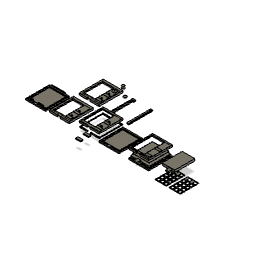
MacroPaw KnGXT (Autodesk Fusion 360 design; units mm, degrees)
Autodesk Fusion 360 part; units mm, degrees
note: some values were not read from the file. Chosen so that the rebuilt part matches the saved one: which bodies a step acts on; which face or edge a step refers to; which pieces of a blend or face edit are solid.
sketch "Sketch1" plane through (0, 0, 0) normal (0, 1, 0) x (1, 0, 0)
  line L0 (-50, -50) -> (44.5, -50)
  line L1 (44.5, -50) -> (44.5, 59)
  line L2 (44.5, 59) -> (-50, 59)
  line L3 (-50, 59) -> (-50, -50)
  dimension "d1" = 94.5
  dimension "d2" = 109
  constraint horizontal L0
  constraint vertical L1
  constraint horizontal L2
  constraint vertical L3
  measures "d1" distance of L0.start L0.end
  measures "d2" distance of L0.start L2.end
extrude "Extrude1" add sketch "Sketch1" along normal blind 1 makes body 1
box "BoxPrimitive1" add length 6 width 15 height 20 placed x (0, 1, 0) y (-1, 0, 0) z (0, 0, 1) at (8.5, 25, 0) separate body makes body 2
move_body "Move1" bodies 2 to x (1, 0, 0) y (0, 1, 0) z (0, 0, 1) at (-3.75, -24, 50)
move_body "Move2" bodies 2 to x (1, 0, 0) y (0, 1, 0) z (0, 0, 1) at (-39.75, 0, 0)
move_body "Move3" bodies 2 to x (1, 0, 0) y (0, 1, 0) z (0, 0, 1) at (35, -1, 0)
copy_body "CopyPasteBodies1" bodies 1 makes body 3
move_body "Move4" bodies 3 to x (1, 0, 0) y (0, 1, 0) z (0, 0, 1) at (0, -10, 0)
copy_body "CopyPasteBodies2" bodies 3 makes body 4
move_body "Move5" bodies 4 to x (1, 0, 0) y (0, 1, 0) z (0, 0, 1) at (0, -10, 0)
move_face "OffsetFaces1" offset -5 1 faces at (-50, -9.6667, -22.6667) on bodies 3
move_face "OffsetFaces2" offset -3 1 faces at (-15.1667, -9.3333, -59) on bodies 3
move_face "OffsetFaces3" offset -5 1 faces at (44.5, -9.3333, -20.6667) on bodies 3
move_face "OffsetFaces4" offset -5 1 faces at (-16.8333, -9.6667, 50) on bodies 3
copy_body "CopyPasteBodies3" bodies 3 makes body 5
move_body "Move6" bodies 5 to x (1, 0, 0) y (0, 1, 0) z (0, 0, 1) at (0, 20, 0)
move_face "OffsetFaces5" offset 3 1 faces at (-16.8333, -10, -22.3333) on bodies 3
copy_body "CopyPasteBodies4" bodies 1 makes body 6
move_body "Move7" bodies 6 to x (1, 0, 0) y (0, 1, 0) z (0, 0, 1) at (0, -10, 0)
move_face "OffsetFaces6" offset 5 1 faces at (13, -19.6667, -59) on bodies 4
move_face "OffsetFaces7" offset 5 1 faces at (-18.5, -19.6667, 50) on bodies 4
move_face "OffsetFaces8" offset 5 1 faces at (-18.5, -19, -24.3333) on bodies 4
move_body "Move8" bodies 4 to x (1, 0, 0) y (0, 1, 0) z (0, 0, 1) at (0, 5, 0)
copy_body "CopyPasteBodies5" bodies 2 makes body 7
move_body "Move9" bodies 7 to x (1, 0, 0) y (0, 1, 0) z (0, 0, 1) at (0, -10, 0)
combine "Combine1" operation cut target body 4 tool bodies 3 6 7
sketch "Sketch3" plane through (0, 1, 0) normal (0, 1, 0) x (-1, 0, 0)
  line L0 (50, -59) -> (50, 50)
  line L1 (50, 50) -> (-44.5, 50)
  line L2 (-44.5, 50) -> (-44.5, -59)
  line L3 (-44.5, -59) -> (50, -59)
  line L4 (-175, 0) -> (-118.9, 0)
  line L5 (-118.9, 0) -> (-118.9, 94.2)
  line L6 (-118.9, 94.2) -> (-175, 94.2)
  line L7 (-175, 94.2) -> (-175, 0)
  dimension "d39" = 56.1
  dimension "d40" = 94.2
  constraint horizontal L4
  constraint vertical L5
  constraint horizontal L6
  constraint vertical L7
  measures "d39" distance of L4.start L4.end
  measures "d40" distance of L4.start L6.end
sketch "Sketch4" plane through (0, 11, 0) normal (0, 1, 0) x (-1, 0, 0)
  line L0 (45, -56) -> (45, 45)
  line L1 (45, 45) -> (-39.5, 45)
  line L2 (-39.5, 45) -> (-39.5, -56)
  line L3 (-39.5, -56) -> (45, -56)
  line L4 (-173, 2) -> (-159, 2)
  line L5 (-159, 2) -> (-159, 16)
  line L6 (-159, 16) -> (-173, 16)
  line L7 (-173, 16) -> (-173, 2)
  line L8 (-173, 21.05) -> (-159, 21.05)
  line L9 (-159, 21.05) -> (-159, 35.05)
  line L10 (-159, 35.05) -> (-173, 35.05)
  line L11 (-173, 35.05) -> (-173, 21.05)
  line L12 (-173, 40.1) -> (-159, 40.1)
  line L13 (-159, 40.1) -> (-159, 54.1)
  line L14 (-159, 54.1) -> (-173, 54.1)
  line L15 (-173, 54.1) -> (-173, 40.1)
  line L16 (-173, 59.15) -> (-159, 59.15)
  line L17 (-159, 59.15) -> (-159, 73.15)
  line L18 (-159, 73.15) -> (-173, 73.15)
  line L19 (-173, 73.15) -> (-173, 59.15)
  line L20 (-173, 78.2) -> (-159, 78.2)
  line L21 (-159, 78.2) -> (-159, 92.2)
  line L22 (-159, 92.2) -> (-173, 92.2)
  line L23 (-173, 92.2) -> (-173, 78.2)
  line L24 (-118.9, 94.2) -> (-175, 94.2)
  line L25 (-153.95, 78) -> (-139.95, 78)
  line L26 (-139.95, 78) -> (-139.95, 92)
  line L27 (-139.95, 92) -> (-153.95, 92)
  line L28 (-153.95, 92) -> (-153.95, 78)
  line L29 (-153.95, 59) -> (-139.95, 59)
  line L30 (-139.95, 59) -> (-139.95, 73)
  line L31 (-139.95, 73) -> (-153.95, 73)
  line L32 (-153.95, 73) -> (-153.95, 59)
  line L33 (-153.95, 40) -> (-139.95, 40)
  line L34 (-139.95, 40) -> (-139.95, 54)
  line L35 (-139.95, 54) -> (-153.95, 54)
  line L36 (-153.95, 54) -> (-153.95, 40)
  line L37 (-153.95, 21) -> (-139.95, 21)
  line L38 (-139.95, 21) -> (-139.95, 35)
  line L39 (-139.95, 35) -> (-153.95, 35)
  line L40 (-153.95, 35) -> (-153.95, 21)
  line L41 (-144.425, 2) -> (-130.425, 2)
  line L42 (-130.425, 2) -> (-130.425, 16)
  line L43 (-130.425, 16) -> (-144.425, 16)
  line L44 (-144.425, 16) -> (-144.425, 2)
  line L45 (-134.9, 78) -> (-120.9, 78)
  line L46 (-120.9, 78) -> (-120.9, 92)
  line L47 (-120.9, 92) -> (-134.9, 92)
  line L48 (-134.9, 92) -> (-134.9, 78)
  line L49 (-134.9, 59) -> (-120.9, 59)
  line L50 (-120.9, 59) -> (-120.9, 73)
  line L51 (-120.9, 73) -> (-134.9, 73)
  line L52 (-134.9, 73) -> (-134.9, 59)
  line L53 (-134.9, 40) -> (-120.9, 40)
  line L54 (-120.9, 40) -> (-120.9, 54)
  line L55 (-120.9, 54) -> (-134.9, 54)
  line L56 (-134.9, 54) -> (-134.9, 40)
  line L57 (-134.9, 21) -> (-120.9, 21)
  line L58 (-120.9, 21) -> (-120.9, 35)
  line L59 (-120.9, 35) -> (-134.9, 35)
  line L60 (-134.9, 35) -> (-134.9, 21)
  dimension "d41" = 14
  dimension "d42" = 14
  dimension "d43" = 14
  dimension "d44" = 14
  dimension "d45" = 14
  dimension "d46" = 14
  dimension "d47" = 14
  dimension "d48" = 14
  dimension "d49" = 14
  dimension "d50" = 14
  dimension "d51" = 2
  dimension "d52" = 19.05
  dimension "d53" = 19.05
  dimension "d54" = 19.05
  dimension "d55" = 19.05
  dimension "d56" = 14
  dimension "d57" = 14
  dimension "d58" = 19.05
  dimension "d59" = 14
  dimension "d60" = 14
  dimension "d61" = 19.05
  dimension "d62" = 14
  dimension "d63" = 14
  dimension "d64" = 19.05
  dimension "d65" = 14
  dimension "d66" = 14
  dimension "d67" = 19.05
  dimension "d68" = 14
  dimension "d69" = 14
  dimension "d70" = 28.575
  dimension "d71" = 14
  dimension "d72" = 14
  dimension "d73" = 19.05
  dimension "d74" = 14
  dimension "d75" = 14
  dimension "d76" = 19.05
  dimension "d77" = 14
  dimension "d78" = 14
  dimension "d79" = 19.05
  dimension "d80" = 19.05
  constraint horizontal L4
  constraint vertical L5
  constraint horizontal L6
  constraint vertical L7
  constraint horizontal L8
  constraint vertical L9
  constraint horizontal L10
  constraint vertical L11
  constraint horizontal L12
  constraint vertical L13
  constraint horizontal L14
  constraint vertical L15
  constraint horizontal L16
  constraint vertical L17
  constraint horizontal L18
  constraint vertical L19
  constraint horizontal L20
  constraint vertical L21
  constraint horizontal L22
  constraint vertical L23
  constraint horizontal L25
  constraint vertical L26
  constraint horizontal L27
  constraint vertical L28
  constraint horizontal L29
  constraint vertical L30
  constraint horizontal L31
  constraint vertical L32
  constraint horizontal L33
  constraint vertical L34
  constraint horizontal L35
  constraint vertical L36
  constraint horizontal L37
  constraint vertical L38
  constraint horizontal L39
  constraint vertical L40
  constraint horizontal L41
  constraint vertical L42
  constraint horizontal L43
  constraint vertical L44
  constraint horizontal L45
  constraint vertical L46
  constraint horizontal L47
  constraint vertical L48
  constraint horizontal L49
  constraint vertical L50
  constraint horizontal L51
  constraint vertical L52
  constraint horizontal L53
  constraint vertical L54
  constraint horizontal L55
  constraint vertical L56
  constraint horizontal L57
  constraint vertical L58
  constraint horizontal L59
  constraint vertical L60
  measures "d41" distance of L4.start L4.end
  measures "d42" distance of L4.start L6.end
  measures "d43" distance of L8.start L8.end
  measures "d44" distance of L8.start L10.end
  measures "d45" distance of L12.start L12.end
  measures "d46" distance of L12.start L14.end
  measures "d47" distance of L16.start L16.end
  measures "d48" distance of L16.start L18.end
  measures "d49" distance of L20.start L20.end
  measures "d50" distance of L20.start L22.end
  measures "d51" distance of L22 L24
  measures "d52" distance of L18 L22
  measures "d53" distance of L14 L18
  measures "d54" distance of L10 L14
  measures "d55" distance of L6 L10
  measures "d56" distance of L25.start L25.end
  measures "d57" distance of L25.start L27.end
  measures "d58" distance of L23 L28
  measures "d59" distance of L29.start L29.end
  measures "d60" distance of L29.start L31.end
  measures "d61" distance of L19 L32
  measures "d62" distance of L33.start L33.end
  measures "d63" distance of L33.start L35.end
  measures "d64" distance of L15 L36
  measures "d65" distance of L37.start L37.end
  measures "d66" distance of L37.start L39.end
  measures "d67" distance of L11 L40
  measures "d68" distance of L41.start L41.end
  measures "d69" distance of L41.start L43.end
  measures "d70" distance of L7 L44
  measures "d71" distance of L45.start L45.end
  measures "d72" distance of L45.start L47.end
  measures "d73" distance of L28 L48
  measures "d74" distance of L49.start L49.end
  measures "d75" distance of L49.start L51.end
  measures "d76" distance of L32 L52
  measures "d77" distance of L53.start L53.end
  measures "d78" distance of L53.start L55.end
  measures "d79" distance of L36 L56
  measures "d80" distance of L40 L60
extrude "Extrude2" add sketch "Sketch3" along normal blind 2 separate body contours L4 L5 L6 L7 makes body 8
extrude "Extrude3" cut sketch "Sketch4" against normal blind 15 contours L4 L5 L6 L7 | L8 L9 L10 L11 | L12 L13 L14 L15 | L16 L17 L18 L19 | L20 L21 L22 L23 | L25 L26 L27 L28 | L29 L30 L31 L32 | L33 L34 L35 L36 | L37 L38 L39 L40 | L41 L42 L43 L44 | L45 L46 L47 L48 | L49 L50 L51 L52 | L53 L54 L55 L56 | L57 L58 L59 L60 bodies 8
copy_body "CopyPasteBodies6" bodies 8 makes body 9
move_body "Move10" bodies 9 to x (1, 0, 0) y (0, 1, 0) z (0, 0, 1) at (70, 0, 0)
move_face "OffsetFaces9" offset -0.25 1 faces at (219.2833, 3, 11.3333) on bodies 9
sketch "Sketch5" plane through (-15, 0, 0) normal (1, 0, 0) x (0, 0, -1)
  line L0 (-55, -9) -> (-55, -10)
  line L1 (-55, -10) -> (-50, -10)
  line L2 (-50, -10) -> (-50, -9)
  line L3 (-50, -9) -> (-55, -9)
move_body "Move11" bodies 2 to x (1, 0, 0) y (0, 1, 0) z (0, 0, 1) at (1.5, 0, 0)
move_face "OffsetFaces10" offset -0.5 2 faces at (0, -9.3333, 51.6667) (14.8333, -9.6667, 50) on bodies 4
extrude "Extrude4" add sketch "Sketch5" along normal blind 1.5 bodies 4
box "BoxPrimitive2" add length 6 width 119 height 3 placed x (0, 1, 0) y (0, 0, -1) z (-1, 0, 0) at (-50, -15, 55) bodies 4
extrude "Extrude5" add 1 faces at (15.1667, -9.6667, 50.5) along direction (0, 0, -1) blind 0.5 on bodies 4 bodies 4
box "BoxPrimitive3" add length 6 width 119 height 3 placed x (0, 1, 0) y (0, 0, 1) z (1, 0, 0) at (44.5, -15, -64) bodies 4
box "BoxPrimitive4" add length 119 width 100.5 height 8 placed x (0, 0, -1) y (-1, 0, 0) z (0, 1, 0) at (47.5, -9, 55) separate body makes body 10
move_body "Move13" bodies 10 to x (1, 0, 0) y (0, 1, 0) z (0, 0, 1) at (0, 9, 0)
combine "Combine2" operation cut target body 10 tool bodies 1 2 keep tools
move_body "Move14" bodies 10 to x (1, 0, 0) y (0, 1, 0) z (0, 0, 1) at (0, 30, 0)
copy_body "CopyPasteBodies8" bodies 5 makes body 11
move_body "Move15" bodies 11 to x (1, 0, 0) y (0, 1, 0) z (0, 0, 1) at (0, 20, 0)
move_body "Move16" bodies 11 to x (1, 0, 0) y (0, 1, 0) z (0, 0, 1) at (150, 0, 0)
extrude "Extrude6" add 1 faces at (133.1667, 31, -22.3333) along direction (0, 1, 0) blind 10 on bodies 11 bodies 11
move_body "Move17" bodies 11 to x (1, 0, 0) y (0, 1, 0) z (0, 0, 1) at (-150, 0, 0)
move_body "Move18" bodies 11 to x (1, 0, 0) y (0, 1, 0) z (0, 0, 1) at (-2.5, 0, 0)
move_body "Move19" bodies 11 to x (1, 0, 0) y (0, 1, 0) z (0, 0, 1) at (0, 0, -2.5)
move_body "Move20" bodies 11 to x (1, 0, 0) y (0, 1, 0) z (0, 0, 1) at (110, 0, 0)
extrude "Extrude7" cut 1 faces at (147, 33.6667, 8.8333) along direction (-1, 0, 0) blind 21 on bodies 11 bodies 11
move_body "Move21" bodies 11 to x (1, 0, 0) y (0, 1, 0) z (0, 0, 1) at (-110, 0, 0)
combine "Combine3" operation cut target body 10 tool bodies 11 keep tools
move_body "Move22" bodies 11 to x (1, 0, 0) y (0, 1, 0) z (0, 0, 1) at (150, 0, 0)
copy_body "CopyPasteBodies9" bodies 2 makes body 12
move_body "Move23" bodies 12 to x (1, 0, 0) y (0, 1, 0) z (0, 0, 1) at (0, 30, -10)
combine "Combine4" operation cut target body 10 tool bodies 12 keep tools
move_body "Move24" bodies 12 to x (1, 0, 0) y (0, 1, 0) z (0, 0, 1) at (150, 0, 0)
move_face "OffsetFaces11" offset -6 1 faces at (35, 31, 11.1667) on bodies 10
extrude "Extrude8" cut 1 faces at (-26.3333, 37.3333, 42.5) along direction (0, 0, 1) blind 4 on bodies 10 bodies 10
extrude "Extrude9" add 1 faces at (39.3333, 37, 11.1667) along direction (0, -1, 0) blind 1 on bodies 10 bodies 10
box "BoxPrimitive5" add length 12 width 26 height 5 placed x (0, 0, -1) y (-1, 0, 0) z (0, 1, 0) at (47.5, 38, 55) separate body makes body 13
move_body "Move25" bodies 13 to x (1, 0, 0) y (0, 1, 0) z (0, 0, 1) at (-5.5, 0, 0)
move_body "Move26" bodies 13 to x (1, 0, 0) y (0, 1, 0) z (0, 0, 1) at (0, 0, -10)
copy_body "CopyPasteBodies10" bodies 13 makes body 14
move_body "Move27" bodies 14 to x (1, 0, 0) y (0, 1, 0) z (0, 0, 1) at (0, 0, -49)
move_body "Move28" bodies 14 to x (1, 0, 0) y (0, 1, 0) z (0, 0, 1) at (0, 0, -0.25)
move_body "Move29" bodies 14 13 to x (1, 0, 0) y (0, 1, 0) z (0, 0, 1) at (0, -5.5, 0)
combine "Combine5" operation cut target body 10 tool bodies 14 13 keep tools
move_body "Move30" bodies 13 14 to x (1, 0, 0) y (0, 1, 0) z (0, 0, 1) at (0, 0, 100)
extrude "Extrude10" add 2 faces at (-19.5, -11, -64) (14, 32.6667, -64) along direction (0, 0, -1) blind 1 on bodies 4 10 bodies 4 10
extrude "Extrude11" add 2 faces at (32.1667, 34.6667, 55) (31.8333, -11.3333, 55) along direction (0, 0, 1) blind 1 on bodies 4 10 bodies 10 4
copy_body "CopyPasteBodies11" bodies 10 4 makes body 15 makes body 16
move_body "Move31" bodies 15 16 to x (1, 0, 0) y (0, 1, 0) z (0, 0, 1) at (-150, 0, 0)
move_body "Move32" bodies 15 to x (1, 0, 0) y (0, 1, 0) z (0, 0, 1) at (0, -39, 0)
extrude "Extrude12" cut 1 faces at (-149.5, -9.3333, 54) along direction (1, 0, 0) blind 1 on bodies 16 bodies 16
extrude "Extrude13" cut 1 faces at (0.5, -9.3333, 54) along direction (1, 0, 0) blind 1 on bodies 4 bodies 4
hole "Hole3" at (-200.5, -15, 53.3) direction (0, 1, 0) diameter 2.75 depth 10 tip angle 180 bodies 15 16
hole "Hole4" at (-105, -15, 53.3) direction (0, 1, 0) diameter 2.75 depth 10 tip angle 180 bodies 15 16
hole "Hole5" at (-105, -15, -62.3) direction (0, 1, 0) diameter 2.75 depth 10 tip angle 180 bodies 15 16
hole "Hole6" at (-200.5, -15, -62.3) direction (0, 1, 0) diameter 2.75 depth 10 tip angle 180 bodies 15 16
move_body "Move33" bodies 15 to x (1, 0, 0) y (0, 1, 0) z (0, 0, 1) at (0, 30, 0)
move_body "Move34" bodies 15 to x (1, 0, 0) y (0, 1, 0) z (0, 0, 1) at (-100, 0, 0)
extrude "Extrude14" add 1 faces at (-297.5, 27.6667, -23.5) along direction (1, 0, 0) blind 3 on bodies 15 bodies 15
extrude "Extrude15" add 1 faces at (-274.3333, 27.6667, -58.5) along direction (0, 0, 1) blind 5 on bodies 15 bodies 15
extrude "Extrude16" add 1 faces at (-254.1667, 28.3333, 46.5) along direction (0, 0, -1) blind 5 on bodies 15 bodies 15
extrude "Extrude17" add 1 faces at (-234, 28.1667, -41.0833) along direction (-1, 0, 0) blind 3 on bodies 15 bodies 15
extrude "Extrude18" cut 1 faces at (-234, 27.5, 43.8333) along direction (-1, 0, 0) blind 3 on bodies 15 bodies 15
extrude "Extrude19" add 2 faces at (-208, 27.5, 41) (-208, 27.5, -12.25) along direction (-1, 0, 0) blind 3 on bodies 15 bodies 15
extrude "Extrude20" add 2 faces at (-219.6667, 28.5, 39.8333) (-228.3333, 28.5, -12.25) along direction (0, -1, 0) blind 1.5 on bodies 15 bodies 15
hole "Hole7" at (-223.5, 29, 23.5) direction (0, -1, 0) diameter 8 depth 10 tip angle 180 bodies 15
hole "Hole8" at (-223.5, 29, -15.75) direction (0, -1, 0) diameter 8 depth 10 tip angle 180 bodies 15
move_body "Move35" bodies 13 14 to x (1, 0, 0) y (0, 1, 0) z (0, 0, 1) at (-250, 0, -100)
move_body "Move36" bodies 13 14 to x (1, 0, 0) y (0, 1, 0) z (0, 0, 1) at (0, -8, 0)
move_body "Move37" bodies 13 to x (1, 0, 0) y (0, 1, 0) z (0, 0, 1) at (5.5, -0.5, 11)
move_body "Move38" bodies 14 to x (1, 0, 0) y (0, 1, 0) z (0, 0, 1) at (5.5, -0.5, 48.25)
move_body "Move39" bodies 13 14 to x (1, 0, 0) y (0, 1, 0) z (0, 0, 1) at (0, 0, -45)
move_body "Move40" bodies 13 to x (1, 0, 0) y (0, 1, 0) z (0, 0, 1) at (-8.5, 0, 29)
move_body "Move41" bodies 13 to x (1, 0, 0) y (0, 1, 0) z (0, 0, 1) at (0, -2, 0)
move_body "Move42" bodies 14 to x (1, 0, 0) y (0, 1, 0) z (0, 0, 1) at (0, -2, 0)
move_body "Move43" bodies 14 to x (1, 0, 0) y (0, 1, 0) z (0, 0, 1) at (-8.5, 0, 0)
move_body "Move44" bodies 14 to x (1, 0, 0) y (0, 1, 0) z (0, 0, 1) at (0, 0, 2)
move_body "Move45" bodies 14 to x (1, 0, 0) y (0, 1, 0) z (0, 0, 1) at (0, 0, -0.25)
move_body "Move46" bodies 14 13 to x (1, 0, 0) y (0, 1, 0) z (0, 0, 1) at (0, 1.75, 0)
move_body "Move47" bodies 14 13 to x (1, 0, 0) y (0, 1, 0) z (0, 0, 1) at (0, -0.25, 0)
move_body "Move48" bodies 13 14 to x (1, 0, 0) y (0, 1, 0) z (0, 0, 1) at (0, 0.15, 0)
combine "Combine6" operation cut target body 15 tool bodies 13 14 keep tools
move_body "Move49" bodies 14 13 to x (1, 0, 0) y (0, 1, 0) z (0, 0, 1) at (0, 0, 100)
ref_plane "WorkPlane1" through (-252.75, 23, -4.5) normal (0, -1, 0) x (0, 0, 1)
split "Split1" by plane through (-252.75, 23, -4.5) normal (0, -1, 0) bodies 15 makes body 17 at (-234.4583, 21, 53.1)
copy_body "CopyPasteBodies12" bodies 17 makes body 18
move_body "Move50" bodies 18 to x (1, 0, 0) y (0, 1, 0) z (0, 0, 1) at (0, -20, 0)
combine "Combine7" operation add target body 17 tool bodies 15
move_face "OffsetFaces12" offset -0.5 1 faces at (-204.283, 1.6667, 54.4733) on bodies 18
move_face "OffsetFaces13" offset -0.5 1 faces at (-300.8393, 1.6667, 51.9675) on bodies 18
move_face "OffsetFaces14" offset -0.5 1 faces at (-300.8393, 1.6667, -63.6325) on bodies 18
move_face "OffsetFaces15" offset -0.5 1 faces at (-205.717, 1.6667, -63.4733) on bodies 18
copy_body "CopyPasteBodies13" bodies 17 18 makes body 19 makes body 20
move_body "Move51" bodies 19 20 to x (1, 0, 0) y (0, 1, 0) z (0, 0, 1) at (-150, 0, 0)
move_face "OffsetFaces16" offset 2 5 faces at (-384.1667, 23, 50) (-355.5, 25, 13.6667) (-437.8333, 23, 50) (-450, 25, -22.6667) (-387, 25, -59) on bodies 19
move_face "OffsetFaces17" offset -1 2 faces at (-384.6229, 1, 53.0484) (-387.6667, 23, -57) on bodies 19 20
move_face "OffsetFaces18" offset 1 1 faces at (-384.8333, 21, 50.6667) on bodies 19
delete_face "DeleteFace1" 18 faces at (-384.6229, 2, 53.0484) (-384.6229, 3, 53.0484) (-383.1667, 2.6667, 56) (-426.6667, 2.3333, 56) (-384.1667, 2.3333, 50) (-355.5, 2.3333, 13.6667) (-450, 2.3333, -22.6667) (-354.2717, 2.3333, -60.5722) (-437.8333, 2.6667, 50) (-386, 2.3333, -65) (-355.7283, 2.3333, 51.5722) (-352.5, 2.3333, -24.6667) (-449.7717, 2.3333, -60.5722) (-387, 2.6667, -59) (-413.5, 2.6667, 52) (-451.2283, 2.3333, 51.5722) (-398.5, 2.6667, 52) (-453, 2.6667, 15.6667) on bodies 20
sketch "Sketch10" plane through (0, 20, 0) normal (0, -1, 0) x (1, 0, 0)
  circle A0 centre (-450.5, -62.3) radius 1.375
  circle A1 centre (-355, -62.3) radius 1.375
  circle A2 centre (-355, 53.3) radius 1.375
  circle A3 centre (-450.5, 53.3) radius 1.375
  line L0 (-413.5, 48) -> (-413.5, 56)
  line L1 (-413.5, 56) -> (-453, 56)
  line L2 (-453, 56) -> (-453, -65)
  line L3 (-453, -65) -> (-352.5, -65)
  line L4 (-352.5, -65) -> (-352.5, 56)
  line L5 (-352.5, 56) -> (-398.5, 56)
  line L6 (-398.5, 56) -> (-398.5, 48)
  line L7 (-398.5, 48) -> (-357.5, 48)
  line L8 (-357.5, 48) -> (-357.5, -58)
  line L9 (-357.5, -58) -> (-448, -58)
  line L10 (-448, -58) -> (-448, 48)
  line L11 (-448, 48) -> (-413.5, 48)
extrude "Extrude21" add sketch "Sketch10" along normal blind 0.5 bodies 19
copy_body "CopyPasteBodies14" bodies 16 makes body 21
move_body "Move52" bodies 21 to x (1, 0, 0) y (0, 1, 0) z (0, 0, 1) at (-250, 0, 0)
extrude "Extrude22" add 1 faces at (-448, 24.5, -22.6667) along direction (1, 0, 0) blind 1 on bodies 19 bodies 19
extrude "Extrude23" add 2 faces at (-384.8333, 22, 48) (-424.6667, 22, 48) along direction (0, 0, -1) blind 1 on bodies 19 bodies 19
extrude "Extrude24" add 1 faces at (-357.5, 22, 12) along direction (-1, 0, 0) blind 1 on bodies 19 bodies 19
extrude "Extrude25" add 1 faces at (-417.5, 24.5, -58) along direction (0, 0, 1) blind 2 on bodies 19 bodies 19
box "BoxPrimitive6" add length 10 width 15 height 2 placed x (0, 0, 1) y (1, 0, 0) z (0, 1, 0) at (-379, 29, -21) separate body makes body 22
copy_body "CopyPasteBodies15" bodies 22 makes body 23
move_body "Move53" bodies 23 to x (1, 0, 0) y (0, 1, 0) z (0, 0, 1) at (0, 0, 40)
move_body "Move54" bodies 23 22 to x (1, 0, 0) y (0, 1, 0) z (0, 0, 1) at (0, -2, 0)
move_body "Move55" bodies 19 22 23 to x (1, 0, 0) y (0, 1, 0) z (0, 0, 1) at (-120, 0, 0)
move_body "Move56" bodies 23 to x (1, 0, 0) y (0, 1, 0) z (0, 0, 1) at (-8, 0, -1)
move_body "Move57" bodies 22 to x (1, 0, 0) y (0, 1, 0) z (0, 0, 1) at (-8, 0, -0.25)
move_body "Move58" bodies 22 23 to x (1, 0, 0) y (0, 1, 0) z (0, 0, 1) at (5, 0, 0)
combine "Combine8" operation add target body 19 tool bodies 23 22
extrude "Extrude26" add 1 faces at (-489.6667, 27.55, -11.25) along direction (0, 0, 1) blind 0.5 on bodies 19 bodies 19
extrude "Extrude27" cut 1 faces at (-489.6667, 27.55, 0.75) along direction (0, 0, 1) blind 0.5 on bodies 19 bodies 19
hole "Hole9" at (-493.5, 29, 23) direction (0, -1, 0) diameter 8 depth 10 tip angle 180 bodies 19
hole "Hole10" at (-493.5, 29, -15) direction (0, -1, 0) diameter 8 depth 10 tip angle 180 bodies 19
box "BoxPrimitive7" add length 6 width 6 height 8 placed x (0, 0, -1) y (1, 0, 0) z (0, -1, 0) at (-478.5, 19.5, 56) separate body makes body 24
move_body "Move59" bodies 24 to x (1, 0, 0) y (0, 1, 0) z (0, 0, 1) at (0, 8, 0)
copy_body "CopyPasteBodies16" bodies 24 makes body 25
move_body "Move60" bodies 25 to x (1, 0, 0) y (0, 1, 0) z (0, 0, 1) at (-94.5, 0, 0)
move_body "Move61" bodies 25 to x (1, 0, 0) y (0, 1, 0) z (0, 0, 1) at (0, 0, -115)
copy_body "CopyPasteBodies17" bodies 24 makes body 26
move_body "Move62" bodies 26 to x (1, 0, 0) y (0, 1, 0) z (0, 0, 1) at (-94.5, 0, 0)
move_body "Move63" bodies 24 to x (1, 0, 0) y (0, 1, 0) z (0, 0, 1) at (0, 0, -115)
copy_body "CopyPasteBodies18" bodies 26 makes body 27
move_body "Move64" bodies 27 to x (1, 0, 0) y (0, 1, 0) z (0, 0, 1) at (94.5, 0, 0)
copy_body "CopyPasteBodies19" bodies 27 makes body 28
move_body "Move65" bodies 28 to x (1, 0, 0) y (0, 1, 0) z (0, 0, 1) at (25.5, -36.5, 0)
move_face "OffsetFaces19" offset -2 1 faces at (-449, -17, 54) on bodies 28
copy_body "CopyPasteBodies20" bodies 28 makes body 29
move_body "Move66" bodies 29 to x (1, 0, 0) y (0, 1, 0) z (0, 0, 1) at (0, 0, -115)
copy_body "CopyPasteBodies21" bodies 29 makes body 30
move_body "Move67" bodies 30 to x (1, 0, 0) y (0, 1, 0) z (0, 0, 1) at (94.5, 0, 0)
copy_body "CopyPasteBodies22" bodies 30 makes body 31
move_body "Move68" bodies 31 to x (1, 0, 0) y (0, 1, 0) z (0, 0, 1) at (0, 0, 115)
combine "Combine9" operation add target body 21 tool bodies 28 31 30 29
combine "Combine10" operation add target body 19 tool bodies 26 27 24 25
move_body "Move69" bodies 19 to x (1, 0, 0) y (0, 1, 0) z (0, 0, 1) at (120, -28.5, 0)
hole "Hole11" at (-449, -15, 52) direction (0, 1, 0) diameter 3 depth 6 tip angle 180 bodies 21
hole "Hole12" at (-449, -15, -61) direction (0, 1, 0) diameter 3 depth 6 tip angle 180 bodies 21
hole "Hole13" at (-356.5, -15, -61) direction (0, 1, 0) diameter 3 depth 6 tip angle 180 bodies 21
hole "Hole14" at (-356.5, -15, 52) direction (0, 1, 0) diameter 3 depth 6 tip angle 180 bodies 21
hole "Hole15" at (-356.5, -15, 52) direction (0, 1, 0) diameter 2.75 depth 12 tip angle 180 bodies 19
hole "Hole16" at (-356.5, -15, -61) direction (0, 1, 0) diameter 2.75 depth 12 tip angle 180 bodies 19
hole "Hole17" at (-449, -15, -61) direction (0, 1, 0) diameter 2.75 depth 12 tip angle 180 bodies 19
hole "Hole18" at (-449, -15, 52) direction (0, 1, 0) diameter 2.75 depth 12 tip angle 180 bodies 19
move_body "Move70" bodies 21 to x (1, 0, 0) y (0, 1, 0) z (0, 0, 1) at (-120, 0, 0)
move_face "OffsetFaces20" offset -0.5 3 faces at (-406.1667, -0.1667, 41.5) (-444.5, -0.1667, 9.8333) (-406.1667, -0.8333, -53.5) on bodies 19
hole "Hole19" at (-372.075, 0.5, -45.025) direction (0, -1, 0) diameter 1 depth 5 tip angle 180 bodies 19
extrude "Extrude28" add 1 faces at (-369.6667, -0.95, -10.75) along direction (0, 0, 1) blind 0.25 on bodies 19 bodies 19
extrude "Extrude29" cut 1 faces at (-369.6667, -0.95, 1.25) along direction (0, 0, 1) blind 0.25 on bodies 19 bodies 19
extrude "Extrude30" cut 1 faces at (-369.6667, -0.95, 28) along direction (0, 0, -1) blind 0.5 on bodies 19 bodies 19
extrude "Extrude31" cut 1 faces at (-369.6667, -0.95, 1.5) along direction (0, 0, 1) blind 0.5 on bodies 19 bodies 19
copy_body "CopyPasteBodies23" bodies 19 makes body 32
move_body "Move71" bodies 32 to x (1, 0, 0) y (0, 1, 0) z (0, 0, 1) at (0, 0, -150)
cylinder "CylinderPrimitive1" add diameter 15 height 1.75 placed x (1, 0, 0) y (0, 0, 1) z (0, -1, 0) at (-372.075, -1.5, -195.025) separate body makes body 33
cylinder "CylinderPrimitive2" add diameter 4 height 7.5 placed x (1, 0, 0) y (0, 0, 1) z (0, -1, 0) at (-372.075, -3.25, -195.025) separate body makes body 34
move_body "Move72" bodies 33 to x (1, 0, 0) y (0, 1, 0) z (0, 0, 1) at (0, 1.75, 0)
combine "Combine11" operation cut target body 32 tool bodies 33 keep tools
move_body "Move73" bodies 33 to x (1, 0, 0) y (0, 1, 0) z (0, 0, 1) at (50, 0, 0)
move_body "Move74" bodies 34 to x (1, 0, 0) y (0, 1, 0) z (0, 0, 1) at (0, 3.75, 0)
combine "Combine12" operation add target body 32 tool bodies 34 keep tools
move_body "Move75" bodies 34 to x (1, 0, 0) y (0, 1, 0) z (0, 0, 1) at (0, -30, 0)
move_body "Move76" bodies 34 to x (1, 0, 0) y (0, 1, 0) z (0, 0, 1) at (50, 28, 0)
copy_body "CopyPasteBodies24" bodies 18 makes body 35
move_body "Move77" bodies 35 to x (1, 0, 0) y (0, 1, 0) z (0, 0, 1) at (-150, -12, -150)
move_face "OffsetFaces21" offset -4 1 faces at (-419.5, -10.3333, -215) on bodies 35
move_face "OffsetFaces22" offset -1 1 faces at (-453, -9.6667, -133) on bodies 35
move_face "OffsetFaces23" offset -4 1 faces at (-439.1667, -10.3333, -94) on bodies 35
move_face "OffsetFaces24" offset -4 1 faces at (-367.8333, -10.3333, -94) on bodies 35
move_face "OffsetFaces25" offset 1 1 faces at (-352.5, -10.3333, -173.3333) on bodies 35
move_face "OffsetFaces26" offset -1 1 faces at (-351.5, -10.3333, -173.3333) on bodies 35
box "BoxPrimitive8" add length 10 width 10 height 5 placed x (0, 0, 1) y (-1, 0, 0) z (0, -1, 0) at (-352.5, -9, -215) separate body makes body 36
copy_body "CopyPasteBodies25" bodies 36 makes body 37
move_body "Move78" bodies 37 to x (1, 0, 0) y (0, 1, 0) z (0, 0, 1) at (-90.5, 0, 0)
copy_body "CopyPasteBodies26" bodies 36 makes body 38
move_body "Move79" bodies 38 to x (1, 0, 0) y (0, 1, 0) z (0, 0, 1) at (0, 0, 111)
copy_body "CopyPasteBodies27" bodies 38 makes body 39
move_body "Move80" bodies 39 to x (1, 0, 0) y (0, 1, 0) z (0, 0, 1) at (-90.5, 0, 0)
combine "Combine13" operation cut target body 35 tool bodies 37 36 38 39 keep tools makes body 40 at (-386.5, -9.6667, -98) makes body 41 at (-354.5, -9, -171.3333) makes body 42 at (-423.3333, -9.6667, -100) makes body 43 at (-452, -9.6667, -137.6667)
move_face "OffsetFaces27" offset 105 1 faces at (-446.3333, -10.6667, -104) on bodies 39
move_face "OffsetFaces28" offset 105 1 faces at (-355.8333, -10.6667, -104) on bodies 38
move_face "OffsetFaces29" offset 5 1 faces at (-443, -10.6667, -208.3333) on bodies 37
extrude "Extrude32" add 1 faces at (-362.5, -10.6667, -208.3333) along direction (-1, 0, 0) blind 5 separate body on bodies 36 makes body 44
copy_body "CopyPasteBodies28" bodies 44 makes body 45
move_body "Move81" bodies 45 to x (1, 0, 0) y (0, 1, 0) z (0, 0, 1) at (0, 0, 111)
copy_body "CopyPasteBodies29" bodies 45 makes body 46
move_body "Move82" bodies 46 to x (1, 0, 0) y (0, 1, 0) z (0, 0, 1) at (-75.5, 0, 0)
copy_body "CopyPasteBodies30" bodies 46 makes body 47
move_body "Move83" bodies 47 to x (1, 0, 0) y (0, 1, 0) z (0, 0, 1) at (24.5, 0, 0)
copy_body "CopyPasteBodies31" bodies 47 makes body 48
move_body "Move84" bodies 48 to x (1, 0, 0) y (0, 1, 0) z (0, 0, 1) at (20, 0, 0)
combine "Combine14" operation cut target body 35 tool bodies 37 44 36 keep tools
combine "Combine15" operation cut target body 42 tool bodies 46 47 keep tools
combine "Combine16" operation cut target body 40 tool bodies 48 45 keep tools
move_body "Move85" bodies 44 36 38 41 45 48 47 46 39 37 to x (1, 0, 0) y (0, 1, 0) z (0, 0, 1) at (150, 0, 0)
move_body "Move86" bodies 43 to x (1, 0, 0) y (0, 1, 0) z (0, 0, 1) at (150, 0, 0)
copy_body "CopyPasteBodies32" bodies 35 42 40 makes body 49 makes body 50 makes body 51
move_body "Move87" bodies 49 50 51 to x (1, 0, 0) y (0, 1, 0) z (0, 0, 1) at (0, 0, 150)
copy_body "CopyPasteBodies33" bodies 49 51 50 makes body 52 makes body 53 makes body 54
move_body "Move88" bodies 52 53 54 to x (1, 0, 0) y (0, 1, 0) z (0, 0, 1) at (-120, 0, 0)
move_body "Move89" bodies 53 54 52 to x (1, 0, 0) y (0, 1, 0) z (0, 0, 1) at (0, 10, 0)
copy_body "CopyPasteBodies34" bodies 34 33 makes body 55 makes body 56
move_body "Move90" bodies 55 56 to x (1, 0, 0) y (0, 1, 0) z (0, 0, 1) at (0, 0, 20)
extrude "Extrude33" add 1 faces at (-323.9076, -1.5, -172.0711) along direction (0, -1, 0) blind 8 on bodies 56 bodies 56 55
move_body "Move91" bodies 56 to x (1, 0, 0) y (0, 1, 0) z (0, 0, 1) at (-50, 0, -20)
move_body "Move92" bodies 56 to x (1, 0, 0) y (0, 1, 0) z (0, 0, 1) at (0, 2, 0)
combine "Combine17" operation cut target body 32 tool bodies 56 keep tools
move_body "Move93" bodies 56 to x (1, 0, 0) y (0, 1, 0) z (0, 0, 1) at (0, 0, -40.5)
copy_body "CopyPasteBodies35" bodies 33 makes body 57
move_body "Move94" bodies 57 to x (1, 0, 0) y (0, 1, 0) z (0, 0, 1) at (-50, 0, 0)
extrude "Extrude34" add 1 faces at (-373.9076, 0.25, -192.0711) along direction (0, 1, 0) blind 0.25 on bodies 57 bodies 57 35 40 42 32
hole "Hole20" at (-372.075, 0.5, -192.025) direction (0, -1, 0) diameter 1 depth 5 tip angle 180 bodies 57
copy_body "CopyPasteBodies36" bodies 33 makes body 58
move_body "Move95" bodies 58 to x (1, 0, 0) y (0, 1, 0) z (0, 0, 1) at (-50, 0.25, 150.5)
move_body "Move98" bodies 58 to x (1, 0, 0) y (0, 1, 0) z (0, 0, 1) at (0, 0, -30)
extrude "Extrude36" add 1 faces at (-373.9076, 0.5, -71.5711) along direction (0, 1, 0) blind 0.25 on bodies 58 bodies 58
move_body "Move99" bodies 58 to x (1, 0, 0) y (0, 1, 0) z (0, 0, 1) at (0, 1.75, 30)
move_body "Move100" bodies 58 to x (1, 0, 0) y (0, 1, 0) z (0, 0, 1) at (0, -2, 0)
combine "Combine18" operation add target body 19 tool bodies 58
copy_body "CopyPasteBodies37" bodies 33 34 makes body 59 makes body 60
move_body "Move101" bodies 59 60 to x (1, 0, 0) y (0, 1, 0) z (0, 0, 1) at (-50, 0.25, 3)
copy_body "CopyPasteBodies38" bodies 59 makes body 61
move_body "Move102" bodies 61 to x (1, 0, 0) y (0, 1, 0) z (0, 0, 1) at (0, -1, 0)
combine "Combine19" operation add target body 57 tool bodies 59
move_body "Move103" bodies 61 to x (1, 0, 0) y (0, 1, 0) z (0, 0, 1) at (0, -20, 0)
move_body "Move104" bodies 61 to x (1, 0, 0) y (0, 1, 0) z (0, 0, 1) at (0, 21, 0)
move_body "Move105" bodies 61 to x (1, 0, 0) y (0, 1, 0) z (0, 0, 1) at (0, -0.25, 0)
move_body "Move106" bodies 60 to x (1, 0, 0) y (0, 1, 0) z (0, 0, 1) at (0, 2, 0)
move_body "Move107" bodies 60 to x (1, 0, 0) y (0, 1, 0) z (0, 0, 1) at (0, -0.25, 0)
extrude "Extrude37" cut 1 faces at (-372.6026, -7, -190.7611) along direction (0, 1, 0) blind 0.25 on bodies 60 bodies 60
combine "Combine20" operation cut target body 57 tool bodies 61
combine "Combine21" operation add target body 57 tool bodies 60
move_face "OffsetFaces30" offset -2.5 1 faces at (-369.6864, -0.3333, -184.9155) on bodies 57
